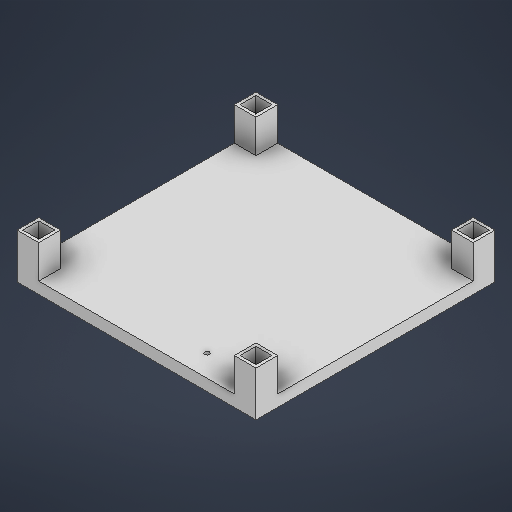
# Autodesk Inventor part: piano inferiore
Saved by Autodesk Inventor 2026.2 (Build 302298000, 298)
## iProperties
Created: 2026-01-19
Part Number: piano inferiore
Material: Generic
Document SubType Name: Modeling
Designer: ASUS
Density: 1 g/cm^3
Appearance: Default
Author: ASUS
Autodesk Inventor part; units mm, degrees
ref_plane "YZ Plane" through (0, 0, 0) normal (1, 0, 0) x (0, 1, 0)
ref_plane "XZ Plane" through (0, 0, 0) normal (0, 1, 0) x (-1, 0, 0)
ref_plane "XY Plane" through (0, 0, 0) normal (0, 0, 1) x (1, 0, 0)
sketch "Sketch1" plane through (0, 0, 0) normal (0, 1, 0) x (-1, 0, 0)
  line L0 (-0.256, 0) -> (-165.256, 0)
  line L1 (-165.256, 0) -> (-165.256, 165)
  line L2 (-165.256, 165) -> (-0.256, 165)
  line L3 (-0.256, 165) -> (-0.256, 0)
  point P0 (0, 0)
  dimension "d0" = 165
  dimension "d1" = 165
  constraints: 8 end point, 2 parallel, 1 horizontal, 1 perpendicular
  measures "d0" distance of L1.end L2.end
  measures "d1" distance of L0.end L1.end
extrude "Extrusion1" add sketch "Sketch1" along normal blind 8
sketch "Sketch2" plane through (0, 8, 0) normal (0, 1, 0) x (1, 0, 0)
  line L0 (165.256, 0) -> (0.256, 0) projected
  line L1 (0.256, 0) -> (15.256, 0)
  line L2 (15.256, 0) -> (15.256, -15)
  line L3 (15.256, -15) -> (0.256, -15)
  line L4 (0.256, -15) -> (0.256, 0)
  line L5 (0.256, -165) -> (165.256, -165) projected
  line L6 (0.256, -165) -> (15.256, -165)
  line L7 (15.256, -165) -> (15.256, -150)
  line L8 (15.256, -150) -> (0.256, -150)
  line L9 (0.256, -150) -> (0.256, -165)
  line L10 (2.256, -152) -> (13.256, -152)
  line L11 (13.256, -152) -> (13.256, -163)
  line L12 (13.256, -163) -> (2.256, -163)
  line L13 (2.256, -163) -> (2.256, -152)
  line L14 (13.256, -13) -> (13.256, -2)
  line L15 (13.256, -2) -> (2.256, -2)
  line L16 (2.256, -2) -> (2.256, -13)
  line L17 (2.256, -13) -> (13.256, -13)
  line L18 (82.756, 0) -> (82.756, -165)
  line L19 (0.256, 0) -> (165.256, 0)
  line L20 (150.256, 0) -> (150.256, -15)
  line L21 (150.256, -15) -> (165.256, -15)
  line L22 (165.256, -15) -> (165.256, 0)
  line L23 (165.256, -165) -> (0.256, -165)
  line L24 (165.256, -165) -> (150.256, -165)
  line L25 (150.256, -165) -> (150.256, -150)
  line L26 (150.256, -150) -> (165.256, -150)
  line L27 (165.256, -150) -> (165.256, -165)
  line L28 (163.256, -152) -> (152.256, -152)
  line L29 (152.256, -152) -> (152.256, -163)
  line L30 (152.256, -163) -> (163.256, -163)
  line L31 (163.256, -163) -> (163.256, -152)
  line L32 (152.256, -13) -> (152.256, -2)
  line L33 (152.256, -2) -> (163.256, -2)
  line L34 (163.256, -2) -> (163.256, -13)
  line L35 (163.256, -13) -> (152.256, -13)
  point P0 (0, 0)
  dimension "d4" = 15
  dimension "d5" = 15
  dimension "d6" = 15
  dimension "d7" = 15
  dimension "d8" = 2
  dimension "d9" = 2
  constraints: 68 end point, 18 symmetric about line, 8 parallel, 4 perpendicular, 2 horizontal, 2 midpoint, 6 other
  measures "d4" distance of L2.end L3.end
  measures "d5" distance of L1.end L2.end
  measures "d6" distance of L8.end L7.end
  measures "d7" distance of L7.end L6.end
  measures "d8" distance between parallel lines of L8 L10
  measures "d9" distance between parallel lines of L2 L14
extrude "Extrusion2" add sketch "Sketch2" along normal blind 23
sketch "Sketch3" plane through (0, 8, 0) normal (0, 1, 0) x (1, 0, 0)
  line L0 (150.256, -150) -> (150.256, -165) projected
  line L1 (0.256, -150) -> (15.256, -150) projected
  line L2 (150.256, -150) -> (15.256, -150)
  line L3 (0.256, -165) -> (165.256, -165) projected
  line L4 (82.756, -165) -> (82.756, -150)
  line L5 (82.756, -150) -> (150.256, -150)
  circle A0 centre (116.506, -150) radius 1.6
  point P0 (0, 0)
  dimension "d12" = 3.2
  constraints: 6 end point, 3 midpoint, 1 centre point, 1 collinear, 1 horizontal
  measures "d12" diameter of A0
extrude "Extrusion3" cut sketch "Sketch3" against normal blind 8 contours A0 L2 | L2 A0
sketch "Sketch4" plane through (0, 0, 0) normal (0, -1, 0) x (1, 0, 0)
  circle A0 centre (116.506, 150) radius 1.6 projected
  circle A1 centre (116.506, 150) radius 2.5
  point P0 (0, 0)
  dimension "d15" = 5
  constraints: 1 centre point, 1 coincident
  measures "d15" diameter of A1
extrude "Extrusion4" cut sketch "Sketch4" against normal blind 3
body "Solid1"
